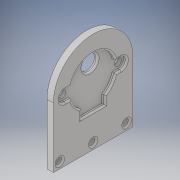
# Autodesk Inventor part: feeder_motor_mount
Saved by Autodesk Inventor 2019 (Build 230136000, 136)
## iProperties
Created: 2018-11-15
Part Number: feeder_motor_mount
Material: Generic
Document SubType Name: Modeling
Designer: chill
Density: 1 g/cm^3
Appearance: Default
Author: chill
Autodesk Inventor part; units mm, degrees
ref_plane "YZ Plane" through (0, 0, 0) normal (1, 0, 0) x (0, 1, 0)
ref_plane "XZ Plane" through (0, 0, 0) normal (0, 1, 0) x (-1, 0, 0)
ref_plane "XY Plane" through (0, 0, 0) normal (0, 0, 1) x (1, 0, 0)
sketch "Sketch1" plane through (0, 0, 0) normal (1, 0, 0) x (0, 1, 0)
  line L0 (0, 25) -> (-38, 25)
  line L1 (0, -25) -> (-38, -25)
  line L2 (-38, 25) -> (-38, -25)
  arc A0 (0, -25) -> (0, 25) centre (0, 0) ccw
  point P0 (0, 0)
  dimension "d3" = 25
  dimension "d4" = 25
  dimension "d7" = 25
  dimension "d9" = 38
  dimension "d10" = 38
  constraints: 6 end point, 2 horizontal, 2 point on circle, 1 centre point, 1 tangent, 1 vertical
  measures "d3" distance from line of L0 point (0, 0)
  measures "d4" distance from line of L1 point (0, 0)
  measures "d7" radius of A0
  measures "d9" distance from line of L2 point (0, 0)
  measures "d10" distance from line of L0.start L2
extrude "Extrusion1" add sketch "Sketch1" along normal blind 4
sketch "Sketch2" plane through (4, 0, 0) normal (1, 0, 0) x (0, 0, -1)
  line L0 (-7.5, -12.2634) -> (-7.5, -17.5)
  line L1 (7.5, -17.5) -> (7.5, -11.9694)
  arc A0 (-17.5, 3.625) -> (-17.5, -3.625) centre (-17.5, 0) ccw
  arc A1 (17.5, -3.625) -> (17.5, 3.625) centre (17.5, 0) ccw
  line L2 (-17.5, 3.625) -> (-13.9104, 3.625)
  line L3 (13.9104, 3.625) -> (17.5, 3.625)
  line L4 (17.5, -3.625) -> (13.9104, -3.625)
  line L5 (-13.9104, -3.625) -> (-17.5, -3.625)
  line L6 (7.5, -17.5) -> (-7.5, -17.5)
  arc A2 (-13.9104, -3.625) -> (-7.5, -12.2634) centre (0, 0) ccw
  arc A3 (7.5, -12.2634) -> (13.9104, -3.625) centre (0, 0) ccw
  arc A4 (13.9104, 3.625) -> (-13.9104, 3.625) centre (0, 0) ccw
  point P0 (-7.5, -15.5)
  point P1 (7.5, -15.5)
  dimension "d14" = 7.5
  dimension "d15" = 7.5
  dimension "d20" = 7.25
  dimension "d21" = 7.25
  dimension "d25" = 90
  dimension "d27" = 0
  dimension "d55" = 13.875
  dimension "d57" = 19.125
  dimension "d58" = 19.125
  dimension "d60" = 14.375
  dimension "d61" = 14.375
  dimension "d62" = 14.375
  dimension "d63" = 3.625
  dimension "d64" = 10
  dimension "d65" = 6.4104
  dimension "d66" = 6.4104
  dimension "d67" = 15.5944
  dimension "d68" = 25
  constraints: 14 end point, 10 point on circle, 5 centre point, 5 tangent, 3 point on line, 2 horizontal, 2 parallel, 1 vertical
  measures "d14" distance from line of point (0, 0) L0
  measures "d15" distance from line of L1 point (0, 0)
  measures "d20" diameter of A0
  measures "d21" diameter of A1
  measures "d25" angle of L1 L4
  measures "d27" distance between parallel lines of L3 L2
  measures "d55" distance between parallel lines of L6 L5
  measures "d57" distance from line of point (7.5, -15.5) L3
  measures "d58" distance from line of point (-7.5, -15.5) L3
  measures "d60" radius of A2
  measures "d61" radius of A3
  measures "d62" radius of A4
  measures "d63" distance from line of point (0, 0) L3
  measures "d64" distance from line of L3.end L1
  measures "d65" distance from line of L3.start L1
  measures "d66" distance from line of L4.end L1
  measures "d67" distance from line of L1.end L3
  measures "d68" distance from line of L2.start L1
extrude "Extrusion2" cut sketch "Sketch2" against normal blind 2
sketch "Sketch3" plane through (2, 0, 0) normal (1, 0, 0) x (0, 0, -1)
  line L0 (-7.5, -17.5) -> (-7.5, -12.2634) projected
  line L1 (7.5, -12.2634) -> (7.5, -17.5) projected
  line L2 (17.5, -3.625) -> (13.9104, -3.625) projected
  arc A0 (17.5, -3.625) -> (17.5, 3.625) centre (17.5, 0) ccw projected
  line L3 (13.9104, 3.625) -> (17.5, 3.625) projected
  line L4 (-17.5, 3.625) -> (-13.9104, 3.625) projected
  arc A1 (-17.5, 3.625) -> (-17.5, -3.625) centre (-17.5, 0) ccw projected
  line L5 (-13.9104, -3.625) -> (-17.5, -3.625) projected
  circle A2 centre (-17.5, 0) radius 2.125
  circle A3 centre (17.5, 0) radius 2.125
  circle A4 centre (0, 8) radius 4.75
  line L6 (7.5, -17.5) -> (-7.5, -17.5) projected
  arc A5 (7.5, -12.2634) -> (13.9104, -3.625) centre (0, 0) ccw projected
  arc A6 (13.9104, 3.625) -> (-13.9104, 3.625) centre (0, 0) ccw projected
  arc A7 (-13.9104, -3.625) -> (-7.5, -12.2634) centre (0, 0) ccw projected
  dimension "d32" = 4.25
  dimension "d33" = 4.25
  dimension "d40" = 9.5
  dimension "d41" = 11.625
  dimension "d42" = 7.5
  constraints: 3 centre point, 2 coincident
  measures "d32" diameter of A2
  measures "d33" diameter of A3
  measures "d40" diameter of A4
  measures "d41" distance from line of A4.centre L2
  measures "d42" distance from line of A4.centre L1
extrude "Extrusion3" cut sketch "Sketch3" against normal through all contours A2 | A3 | A4
sketch "Sketch4" plane through (4, 0, 0) normal (1, 0, 0) x (0, 0, -1)
  circle A0 centre (-21, -34) radius 2
  circle A1 centre (0, -34) radius 2
  circle A2 centre (21, -34) radius 2
  line L0 (-25, -38) -> (25, -38) projected
  line L1 (-25, 0) -> (-25, -38) projected
  line L2 (25, -38) -> (25, 0) projected
  point P0 (0, 0)
  dimension "d43" = 4
  dimension "d44" = 4
  dimension "d45" = 4
  dimension "d46" = 4
  dimension "d47" = 4
  dimension "d48" = 4
  dimension "d49" = 4
  dimension "d50" = 4
  dimension "d51" = 25
  constraints: 3 centre point
  measures "d43" diameter of A0
  measures "d44" diameter of A1
  measures "d45" diameter of A2
  measures "d46" distance from line of L0 A0.centre
  measures "d47" distance from line of L1 A0.centre
  measures "d48" distance from line of L2 A2.centre
  measures "d49" distance from line of L0 A2.centre
  measures "d50" distance from line of L0 A1.centre
  measures "d51" distance from line of A1.centre L2
extrude "Extrusion4" cut sketch "Sketch4" against normal through all
fillet "Fillet1" radius 1 3 edges at (4, -34, 23) (4, -34, 2) (4, -34, -19)
fillet "Fillet2" radius 1 13 edges at (4, 14.375, 0) (4, -8.5664, -11.5437) (4, 0, -21.125) (4, 3.625, -15.7052) (4, -3.625, -15.7052) (4, 0, 21.125) (4, 3.625, 15.7052) (4, -3.625, 15.7052) (4, -8.5664, 11.5437) (4, -17.5, 0) (4, -14.8817, 7.5) (4, -14.8817, -7.5) (2, 8, 4.75)
body "Solid1"
